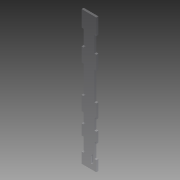
# Autodesk Inventor part: Right_wall
Saved by Autodesk Inventor 2015 (Build 190159000, 159)
## iProperties
Created: 2015-06-19
Part Number: Right_wall
Material: Generic
Document SubType Name: Modeling
Designer: Openlab
Density: 1 g/cm^3
Appearance: Polycarbonate - Clear
Author: Openlab
Autodesk Inventor part; units mm, degrees
ref_plane "YZ Plane" through (0, 0, 0) normal (1, 0, 0) x (0, 1, 0)
ref_plane "XZ Plane" through (0, 0, 0) normal (0, 1, 0) x (-1, 0, 0)
ref_plane "XY Plane" through (0, 0, 0) normal (0, 0, 1) x (1, 0, 0)
sketch "Sketch1" plane through (0, 0, 0) normal (0, 1, 0) x (-1, 0, 0)
  line L0 (21, -23) -> (18.25, -23)
  line L1 (21, -46) -> (18.25, -46)
  line L2 (21, -141) -> (18.25, -141)
  line L3 (21, -66) -> (18.25, -66)
  line L4 (21, -126) -> (18.25, -126)
  line L5 (21, -106) -> (18.25, -106)
  line L6 (2.75, -66) -> (0, -66)
  line L7 (2.75, -106) -> (0, -106)
  line L8 (2.75, -126) -> (0, -126)
  line L9 (2.75, -141) -> (0, -141)
  line L10 (2.75, -46) -> (0, -46)
  line L11 (2.75, -23) -> (0, -23)
  line L12 (21, -156) -> (21, -141)
  line L13 (21, -126) -> (21, -106)
  line L14 (21, -66) -> (21, -46)
  line L15 (21, -23) -> (21, 0)
  line L16 (0, -156) -> (0, -141)
  line L17 (0, -126) -> (0, -106)
  line L18 (0, -66) -> (0, -46)
  line L19 (0, -23) -> (0, 0)
  line L20 (18.25, -141) -> (18.25, -126)
  line L21 (18.25, -106) -> (18.25, -66)
  line L22 (18.25, -46) -> (18.25, -23)
  line L23 (2.75, -141) -> (2.75, -126)
  line L24 (2.75, -106) -> (2.75, -66)
  line L25 (2.75, -46) -> (2.75, -23)
  line L26 (21, -66) -> (21, -46) construction
  line L27 (21, 0) -> (0, 0)
  line L28 (10.5, -68) -> (10.5, -97) construction
  line L29 (18.25, -156) -> (18.25, -176)
  line L30 (18.25, -176) -> (21, -176)
  line L31 (21, -176) -> (21, -191)
  line L32 (21, -191) -> (0, -191)
  line L33 (0, -191) -> (0, -176)
  line L34 (0, -176) -> (2.75, -176)
  line L35 (2.75, -156) -> (2.75, -176)
  line L36 (21, -156) -> (18.25, -156)
  line L37 (2.75, -156) -> (0, -156)
  line L38 (7.55, -174) -> (5.75, -174)
  line L39 (5.75, -174) -> (5.75, -184)
  line L40 (5.75, -184) -> (7.55, -184)
  line L41 (7.55, -184) -> (7.55, -174)
  dimension "d7" = 23
  dimension "d8" = 20
  dimension "d9" = 40
  dimension "d10" = 20
  dimension "d11" = 15
  dimension "d28" = 15.5
  dimension "d31" = 2.75
  dimension "d42" = 23
  dimension "d44" = 15
  dimension "d45" = 20
  dimension "d47" = 15
  dimension "d48" = 7
  dimension "d49" = 1.8
  dimension "d51" = 10
  dimension "d53" = 3
  constraints: 85 end point, 29 collinear, 11 perpendicular, 4 parallel, 4 vertical, 2 point on line, 1 horizontal, 1 other
  measures "d7" distance between parallel lines of L1 L0
  measures "d8" distance between parallel lines of L3 L1
  measures "d9" distance between parallel lines of L5 L3
  measures "d10" distance between parallel lines of L4 L5
  measures "d11" distance between parallel lines of L2 L4
  measures "d28" distance between parallel lines of L23 L20
  measures "d31" distance between parallel lines of L22 L15
  measures "d42" distance from line of L0.start L27
  measures "d44" distance of L30.end L31.end
  measures "d45" distance of L29.start L29.end
  measures "d47" distance of L12.start L2.start
  measures "d48" distance between parallel lines of L40 L32
  measures "d49" distance of L38.start L38.end
  measures "d51" distance of L40.end L38.start
  measures "d53" distance between parallel lines of L35 L39
extrude "Extrusion3" add sketch "Sketch1" along normal blind 3
body "Solid3"
